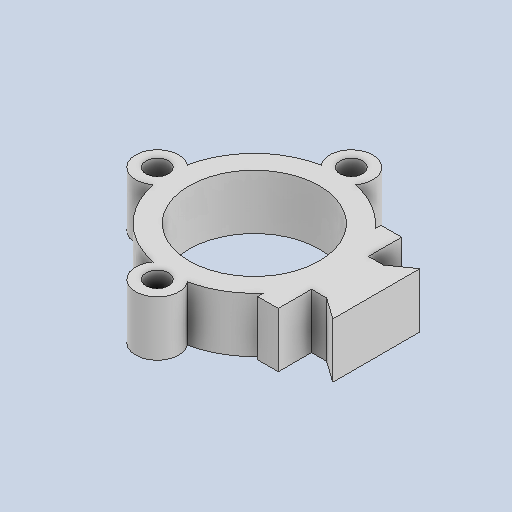
# Autodesk Inventor part: acople_v2
Saved by Autodesk Inventor 2024 (Build 280153000, 153)
## iProperties
Created: 2025-05-21
Part Number: acople_v2
Material: Genérico
Document SubType Name: Modeling
Designer: ANDRES
Density: 1 g/cm^3
Appearance: Valor por defecto
Author: ANDRES
## iProperties of the stored document acople_v2_3DPrint.ipt
Created: 2025-05-21
Part Number: acople_v2_3DPrint
Material: Genérico
Document SubType Name: Modeling
Designer: ANDRES
Density: 1 g/cm^3
Appearance: Valor por defecto
Author: ANDRES
Autodesk Inventor part; units mm, degrees
ref_plane "YZ Plane" through (0, 0, 0) normal (1, 0, 0) x (0, 1, 0)
ref_plane "XZ Plane" through (0, 0, 0) normal (0, 1, 0) x (-1, 0, 0)
ref_plane "XY Plane" through (0, 0, 0) normal (0, 0, 1) x (1, 0, 0)
sketch "Boceto1" plane through (0, 0, 0) normal (0, 1, 0) x (-1, 0, 0)
  line L0 (0, 6.35) -> (0, -6.35)
  line L1 (3.1, 4.15) -> (3.1, -4.15)
  line L2 (0, 6.35) -> (3.1, 4.15)
  line L3 (3.1, -4.15) -> (0, -6.35)
  line L4 (3.1, 4.15) -> (5.3, 4.15)
  line L5 (-4.6452, 0) -> (17.8, 0) construction
  line L6 (3.1, -4.15) -> (5.3, -4.15)
  line L7 (5.3, 9) -> (5.3, -9)
  line L8 (5.3, 9) -> (8.3, 9)
  line L9 (8.3, 9) -> (8.3, -9)
  line L10 (8.3, -9) -> (5.3, -9)
  line L11 (5.3, -9) -> (5.3, 9)
  circle A0 centre (17.8, 0) radius 9.5
  circle A1 centre (17.8, 0) radius 12.5
  circle A2 centre (31.95, 0) radius 1.65
  circle A3 centre (31.95, 0) radius 3.15
  circle A4 centre (17.8, 14.15) radius 3.15
  circle A5 centre (17.8, 14.15) radius 1.65
  circle A6 centre (17.8, -14.15) radius 3.15
  circle A7 centre (17.8, -14.15) radius 1.65
  point P0 (0, 0)
  point P1 (0, 0)
  point P2 (3.1, 0)
  point P3 (5.3, 0)
  point P4 (5.3, 0)
  point P5 (30.3, 0)
  point P6 (17.8, -12.5)
  point P7 (17.8, 12.5)
  point P8 (30.0456, 2.5091)
  point P9 (20.3091, 12.2456)
  point P10 (15.2909, 12.2456)
  point P11 (8.3, 8.124)
  point P12 (8.3, -8.124)
  point P13 (15.2909, -12.2456)
  point P14 (20.3091, -12.2456)
  point P15 (30.0456, -2.5091)
  dimension "d0" = 12.7
  dimension "d1" = 8.3
  dimension "d2" = 3.1
  dimension "d3" = 2.2
  dimension "d4" = 18
  dimension "d5" = 3
  dimension "d6" = 19
  dimension "d7" = 25
  dimension "d8" = 3.3
  dimension "d9" = 6.3
  dimension "d12" = 90
  dimension "d16" = 90
  constraints: 24 end point, 8 centre point, 6 coincident, 4 horizontal, 4 horizontal alignment, 4 midpoint, 4 point on circle, 3 vertical, 2 parallel, 1 concentric, 1 perpendicular, 1 point on line, 1 symmetric about line, 1 tangent, 10 other
  measures "d0" distance of L0.start L0.end
  measures "d1" distance of L1.start L1.end
  measures "d2" distance between parallel lines of L0 L1
  measures "d3" distance of L1.start L4.end
  measures "d4" distance of L7.start L7.end
  measures "d5" distance of L9.end L10.end
  measures "d6" diameter of A0
  measures "d7" diameter of A1
  measures "d8" diameter of A2
  measures "d9" diameter of A3
extrude "Extrusión1" add sketch "Boceto1" along normal blind 8
